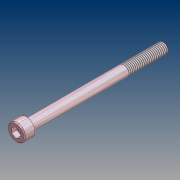
# Autodesk Inventor part: SCREW, SOCKET HD, P, 12.9, M6X1.0X70MM
Saved by Autodesk Inventor 2022.4 (Build 264492000, 492)
## iProperties
Manager: 100-05672
Category: _
Created: 2013-03-06
Material: Generic
Document SubType Name: Modeling
Checked By: 0000586329
Engr Approved By: R
User Status: Released
Description: SCREW, SOCKET HD, P, 12.9, M6X1.0X70MM
Mass: 2.37689 g
Surface Area: 16.984 cm^2
Volume: 2.37689 cm^3
Density: 1 g/cm^3
Designer: keithl , Keith
Mfg Approved By: Keith.Leroux
Appearance: Glossy - Black
Part Number: SCREW, SOCKET HD, P, 12.9, M6X1.0X70MM
Control State: 0
Master: False
Checked Out: False
Shininess: 64.0
CN_SERVICEABLE: _
FIRST_DESCRIPTION: -
PTC_WM_ITERATION: 2
PTC_WM_ORGANIZATION_ID: CLWC
PTC_WM_LIFECYCLE: CLWC_CAD_LC
CN_MASS: 0.002377
CL_runCount: 1
FinishProperty: ToBeSet
SECOND_DESCRIPTION: _
THIRD_DESCRIPTION: _
CN_MFG_PART_NUM: _
CUSTOMERNUMBER: _
Density: 0.0
Volumn: 0.0
Area: 0.0
PropertySet Name: Model Information
Revision Number: A
Author: -
Keywords: -
Subject: _
Autodesk Inventor part; units mm, degrees
ref_plane "YZ Plane" through (0, 0, 0) normal (1, 0, 0) x (0, 1, 0)
ref_plane "XZ Plane" through (0, 0, 0) normal (0, 1, 0) x (-1, 0, 0)
ref_plane "XY Plane" through (0, 0, 0) normal (0, 0, 1) x (1, 0, 0)
sketch "Sketch1" plane through (0, 0, 0) normal (0, 0, 1) x (1, 0, 0)
  circle A0 centre (0, 0) radius 3
  dimension "Diameter" = 6
  constraints: 1 centre point
  measures "Diameter" diameter of A0
extrude "Extrusion1" add sketch "Sketch1" along normal blind 70
sketch "Sketch2" plane through (0, 0, 70) normal (0, 0, 1) x (1, 0, 0)
  circle A0 centre (0, 0) radius 3 projected
  circle A1 centre (0, 0) radius 5
  dimension "Head_Diameter" = 10
  constraints: 1 centre point, 1 coincident
  measures "Head_Diameter" diameter of A1
extrude "Extrusion2" add sketch "Sketch2" along normal blind 6 contours A0 | A1
sketch "Sketch3" plane through (0, 0, 76) normal (0, 0, 1) x (1, 0, 0)
  circle A0 centre (0, 0) radius 5 projected
  circle A1 centre (0, 0) radius 2.8868 construction
  line L0 (0, 2.8868) -> (2.5, 1.4434)
  line L1 (2.5, -1.4434) -> (2.5, 1.4434)
  line L2 (0, 2.8868) -> (-2.5, 1.4434)
  line L3 (-2.5, -1.4434) -> (-2.5, 1.4434)
  line L4 (-2.5, -1.4434) -> (0, -2.8868)
  line L5 (2.5, -1.4434) -> (0, -2.8868)
  dimension "Hex_Width" = 5
  constraints: 12 end point, 6 point on circle, 3 equal length, 1 centre point, 1 coincident, 1 parallel, 1 vertical
  measures "Hex_Width" distance between parallel lines of L0 L4
extrude "Extrusion3" cut sketch "Sketch3" against normal blind 3 contours L0 L1 L5 L4 L3 L2
thread "Thread1" size "M6x1" class "4g6g" standard "ANSI Metric M Profile" length 24
chamfer "Chamfer1" distance 0.6 angle 45 2 edges at (-5, 0, 76) (-3, 0, 0)
equation "\"d9\" = ThreadLength"
equation "\"d12\" = Chamfer"
equation "\"ThreadLength\" = 24"
equation "\"Chamfer\" = 0.6"
body "Solid1"
